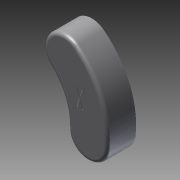
# Autodesk Inventor part: X Button
Saved by Autodesk Inventor 2012 SP1 (Build 160190100, 190)
## iProperties
Created: 2011-12-08
Part Number: X Button
Material: Default
Document SubType Name: Modeling
Designer: 133098
Density: 1 g/cm^3
Author: 133098
Autodesk Inventor part; units mm, degrees
ref_plane "YZ Plane" through (0, 0, 0) normal (1, 0, 0) x (0, 1, 0)
ref_plane "XZ Plane" through (0, 0, 0) normal (0, 1, 0) x (-1, 0, 0)
ref_plane "XY Plane" through (0, 0, 0) normal (0, 0, 1) x (1, 0, 0)
sketch "Sketch1" plane through (0, 0, 0) normal (0, 0, 1) x (1, 0, 0)
  arc A0 (53.8057, 7.6214) -> (60.8401, 7.187) centre (57.3363, 7.6214) ccw
  arc A1 (55.1426, 20.9078) -> (50.5197, 15.5843) centre (52.9772, 18.1193) ccw
  arc A2 (53.8057, 7.6214) -> (50.5197, 15.5843) centre (42.9913, 7.8181) ccw
  arc A3 (60.8401, 7.187) -> (55.1426, 20.9078) centre (45.9242, 9.0366) ccw
  dimension "d3" = 7.0612
  dimension "d4" = 7.0612
  constraints: 10 point on circle, 4 centre point, 3 tangent
  measures "d3" diameter of A0
  measures "d4" diameter of A1
extrude "Extrusion1" add sketch "Sketch1" along normal blind 5.08
fillet "Fillet1" radius 0.635 4 edges at (57.1187, 4.0975, 5.08) (50.3114, 20.4341, 5.08) (52.9896, 11.9441, 5.08) (59.8052, 14.8006, 5.08)
sketch "Sketch2" plane through (0, 0, 5.08) normal (0, 0, 1) x (1, 0, 0)
  line L0 (55.3489, 14.773) -> (60.8716, 14.773) construction
  line L1 (60.8716, 14.773) -> (60.8716, 8.0828) construction
  line L2 (60.8716, 8.0828) -> (55.3489, 8.0828) construction
  line L3 (55.3489, 8.0828) -> (55.3489, 14.773) construction
  line L4 (56.5567, 11.725) -> (56.3245, 11.725)
  line L5 (56.3245, 11.725) -> (55.954, 12.9378)
  line L6 (55.954, 12.9378) -> (55.5761, 11.725)
  line L7 (55.5761, 11.725) -> (55.3563, 11.725)
  line L8 (55.3563, 11.725) -> (55.8429, 13.2514)
  line L9 (55.8429, 13.2514) -> (55.3711, 14.773)
  line L10 (55.3711, 14.773) -> (55.6033, 14.773)
  line L11 (55.6033, 14.773) -> (55.9664, 13.58)
  line L12 (55.9664, 13.58) -> (56.3369, 14.773)
  line L13 (56.3369, 14.773) -> (56.5567, 14.773)
  line L14 (56.5567, 14.773) -> (56.0775, 13.2712)
  line L15 (56.0775, 13.2712) -> (56.5567, 11.725)
  point P0 (0, 0)
  constraints: 2 other
extrude "Extrusion2" cut sketch "Sketch2" against normal blind 0.0635
body "Solid1"
